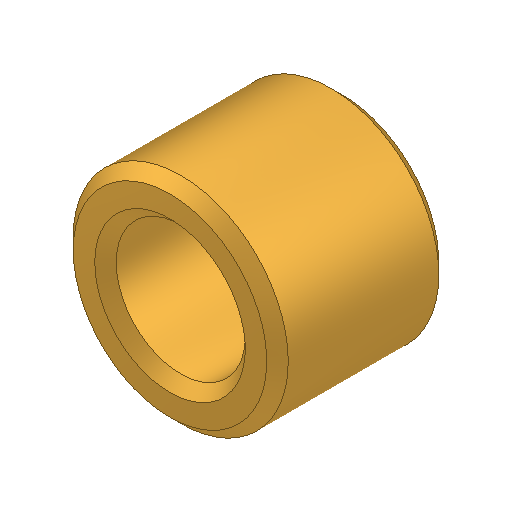
# Autodesk Inventor part: GRJ-03-117
Saved by Autodesk Inventor 2026.1 (Build 301233000, 233)
## iProperties
Company: Gree
Created: 2025-08-15
Part Number: GRJ-03-117
Material: Latão YL
Document SubType Name: Modeling
Designer: Willian Pinheiro
Density: 8.47 g/cm^3
Appearance: Latão - Acetinado
Mass: 3.29955 g
Surface Area: 4.7321 cm^2
Volume: 0.389557 cm^3
Description: Bucha Eixo Ø6
Project: GRJ-03
Checked By: Antonio Lucas
Engr Approved By: Antonio Lucas
Mfg Approved By: Anderson Oliveira
Dimensões: Ø10 x 8 mm
Total: 2
Author: Willian Pinheiro
Title: Soldagem
Revision Number: 00
Autodesk Inventor part; units mm, degrees
ref_plane "YZ Plane" through (0, 0, 0) normal (1, 0, 0) x (0, 1, 0)
ref_plane "XZ Plane" through (0, 0, 0) normal (0, 1, 0) x (-1, 0, 0)
ref_plane "XY Plane" through (0, 0, 0) normal (0, 0, 1) x (1, 0, 0)
sketch "Esboço1" plane through (0, 0, 0) normal (0, 0, 1) x (1, 0, 0)
  line L0 (-6, 0) -> (1, 0) construction
  line L1 (0, -5.6) -> (0, 5.6) construction
  line L2 (-5, 4) -> (-3, 4)
  line L3 (-3, 4) -> (-3, -4)
  line L4 (-3, -4) -> (-5, -4)
  line L5 (-5, -4) -> (-5, 4)
  point P0 (0, 0)
  dimension "d1" = 8
  dimension "d2" = 10
  dimension "d3" = 6
  constraints: 8 end point, 2 parallel, 1 horizontal, 1 perpendicular, 1 other
  measures "d1" distance between parallel lines of L2 L4
  measures "d2" diameter of L5 L1
  measures "d3" diameter of L3 L1
revolve "Revolução1" add sketch "Esboço1" angle 360 about axis through (0, -10, 0) along (0, 1, 0)
chamfer "Chanfro1" distance 0.5 angle 45 4 edges at (5, -4, 0) (3, -4, 0) (3, 4, 0) (5, 4, 0)
